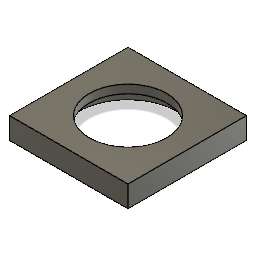
Block (Autodesk Fusion 360 design; units mm, degrees)
Autodesk Fusion 360 part; units mm, degrees
sketch "Sketch1" plane through (0, 0, 0) normal (0, 1, 0) x (1, 0, 0)
  line L0 (-1.375, -1.375) -> (1.375, -1.375)
  line L1 (1.375, -1.375) -> (1.375, 1.375)
  line L2 (1.375, 1.375) -> (-1.375, 1.375)
  line L3 (-1.375, 1.375) -> (-1.375, -1.375)
  line L4 (-1.375, -1.375) -> (1.375, 1.375) construction
  line L5 (1.375, -1.375) -> (-1.375, 1.375) construction
  dimension "d1" = 2.75
  dimension "d2" = 2.75
extrude "Extrude1" add sketch "Sketch1" along normal blind 0.5
ref_plane "WorkPlane1" through (0, 0.25, 0) normal (0, 0, 1) x (1, 0, 0)
sketch "Sketch2" plane through (0, 0.25, 0) normal (0, 0, 1) x (1, 0, 0)
  line L0 (-1.375, -0.25) -> (1.375, -0.25)
  line L1 (0, -0.25) -> (-1.15, -0.25)
  line L2 (-1.375, 0.25) -> (1.375, 0.25)
  line L3 (0, 0.25) -> (0, -0.25)
  line L4 (-1.15, -0.25) -> (-1.15, 0.05)
  line L5 (-1.15, 0.05) -> (-0.9, 0.05)
  line L6 (-0.9, 0.05) -> (-0.8922, 0.25)
  dimension "d5" = 1.15
  dimension "d6" = 0.3
  dimension "d7" = 0.25
  measures "d6" distance of origin
sketch "Sketch3" plane through (0, 0, 0) normal (0, 0, 1) x (1, 0, 0)
revolve "Revolve1" cut sketch "Sketch2" angle 360 about axis through (0, 0.5, 0) along (0, -1, 0)
